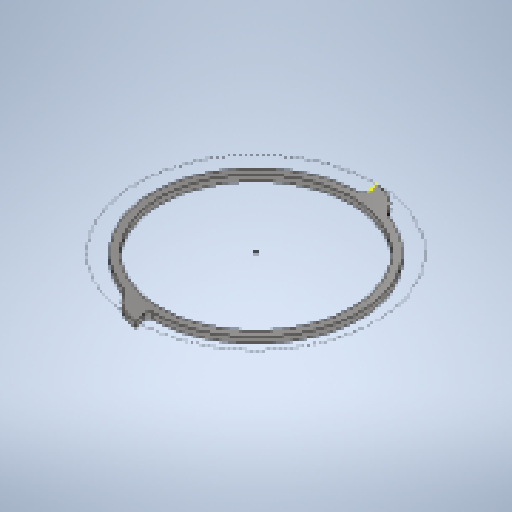
# Autodesk Inventor part: Blade - Ring
Saved by Autodesk Inventor 2023.2 (Build 272271000, 271)
## iProperties
Created: 2023-10-14
Part Number: Blade - Ring
Material: Steel, Mild
Document SubType Name: Modeling
Designer: Nathan Cai
Mass: 134.875 g
Surface Area: 121.592 cm^2
Volume: 17.1815 cm^3
Density: 7.85 g/cm^3
Appearance: Semi-Polished
Author: Nathan Cai
Autodesk Inventor part; units mm, degrees
ref_plane "YZ Plane" through (0, 0, 0) normal (1, 0, 0) x (0, 1, 0)
ref_plane "XZ Plane" through (0, 0, 0) normal (0, 1, 0) x (-1, 0, 0)
ref_plane "XY Plane" through (0, 0, 0) normal (0, 0, 1) x (1, 0, 0)
sketch "Sketch1" plane through (0, 0, 0) normal (0, 1, 0) x (-1, 0, 0)
  circle A0 centre (0, 0) radius 76.2
  circle A1 centre (0, 0) radius 82.55
  line L0 (0, 0) -> (0, -82.55) construction
  line L1 (0, -95.25) -> (-3.422, -82.479)
  arc A2 (-25.4, -78.5452) -> (0, -95.25) centre (0, -67.587) ccw
  line L2 (0, 95.25) -> (3.422, 82.479)
  arc A3 (25.4, 78.5452) -> (0, 95.25) centre (0, 67.587) ccw
  point P0 (0, 82.55)
  point P1 (25.4, 78.5452)
  dimension "d0" = 152.4
  dimension "d1" = 6.35
  dimension "d4" = 15
  dimension "d5" = 12.7
  dimension "d6" = 25.4
  dimension "d9" = 360
  constraints: 7 point on circle, 6 end point, 4 centre point, 2 coincident, 1 line through centre, 1 point on line, 1 vertical, 15 other
  measures "d0" diameter of A0
  measures "d1" radial gap between concentric circles of A0 A1
  measures "d4" angle of L0 L1
  measures "d5" distance of L0.end L1.start
  measures "d6" distance from line of L0 A2.start
extrude "Extrusion1" add sketch "Sketch1" along normal blind 4.7625
fillet "Fillet1" radius 3.175 4 edges at (25.4, 2.3813, -78.5452) (3.422, 2.3813, -82.479) (-25.4, 2.3813, 78.5452) (-3.422, 2.3813, 82.479)
sketch "Sketch2" plane through (0, 4.7625, 0) normal (0, 1, 0) x (1, 0, 0)
  line L0 (0, 95.25) -> (2.3329, 86.5436) projected
  circle A0 centre (0, 0) radius 95.25 construction
  constraints: 1 coincident, 1 vertical alignment, 2 other
body "Solid1"
